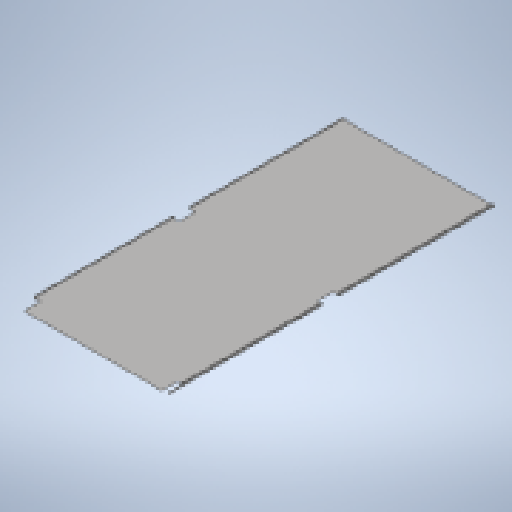
# Autodesk Inventor part: MSC 0101 sheet gills
Saved by Autodesk Inventor 2025 (Build 290162010, 162A)
## iProperties
Created: 2024-06-15
Part Number: MSC 0101 sheet gills
Material: Stainless Steel
Document SubType Name: Sheet Metal
Designer: pokla
Density: 8 g/cm^3
Sheet Metal Rule: Default_mm
Appearance: Default
Stock Number: МОО 0101 лист жабра
Mass: 7357.89 g
Surface Area: 36818.7 cm^2
Volume: 919.736 cm^3
Flat Pattern Width: 96.1524 cm
Flat Pattern Length: 200 cm
Flat Pattern Area: 19230.5 cm^2
Sheet Metal Width: 961,524 mm
Sheet Metal Length: 2000,000 mm
Sheet Metal Area: 1923047,787 mm^2
Author: pokla
Autodesk Inventor part; units mm, degrees
ref_plane "YZ Plane" through (0, 0, 0) normal (1, 0, 0) x (0, 1, 0)
ref_plane "XZ Plane" through (0, 0, 0) normal (0, 1, 0) x (-1, 0, 0)
ref_plane "XY Plane" through (0, 0, 0) normal (0, 0, 1) x (1, 0, 0)
sketch "Sketch6" plane through (0, 0, 0) normal (0, 1, 0) x (-1, 0, 0)
  line L0 (462.5, -1000) -> (-462.5, -1000)
  line L1 (-462.5, -1000) -> (-462.5, 1000)
  line L2 (-462.5, 1000) -> (462.5, 1000)
  line L3 (462.5, 1000) -> (462.5, -1000)
  line L4 (462.5, -1000) -> (-462.5, 1000) construction
  line L5 (-462.5, -1000) -> (462.5, 1000) construction
  point P0 (0, 0)
  dimension "d52" = 925
  dimension "d53" = 2000
  measures "d52" distance of L1.end L2.end
  measures "d53" distance of L0.end L1.end
extrude "Plate2" add sketch "Sketch6" along normal blind 0.5
sketch "Sketch10" plane through (-462, 0, 1000) normal (-1, 0, 0) x (0, -1, 0)
  line L0 (0, -2000) -> (0, 0)
  line L1 (0, 0) -> (-10, 0)
  line L2 (-10, 0) -> (-10, -2000)
  line L3 (-10, -2000) -> (0, -2000)
  constraints: 6 end point, 1 horizontal, 1 perpendicular, 1 vertical
edge flange "Flange1" height 10 angle 90 thickness 0.5 bend radius 0.5 thickness toward (-1, 0, 0) relief straight relief width 0.5 relief depth 0.25 corner gap 0.5 corner form 0 edges at (-462.5, 0.5, 0) (462.5, 0.5, 0) wall of the first edge with corners at (-462, 0, -1000) (-462, 0, 1000) (-462, 10, 1000) (-462, 10, -1000)
bend "Bend2"
corner "Corner2"
sketch "Sketch11" plane through (462.5, 9.5, -1000) normal (0, 1, 0) x (-1, 0, 0)
  line L0 (0, 2000) -> (0, 0)
  line L1 (0, 0) -> (10, 0)
  line L2 (10, 0) -> (10, 2000)
  line L3 (10, 2000) -> (0, 2000)
  constraints: 6 end point, 1 horizontal, 1 perpendicular, 1 vertical
edge flange "Flange2" height 10 angle 90 thickness 0.5 bend radius 0.5 thickness toward (0, 1, 0) relief straight relief width 0.5 relief depth 0.25 corner gap 0.5 corner form 0 edges at (462, 10, 0) (-462, 10, 0) wall of the first edge with corners at (462.5, 9.5, 1000) (462.5, 9.5, -1000) (452.5, 9.5, -1000) (452.5, 9.5, 1000)
bend "Bend3"
corner "Corner3"
sketch "Sketch12" plane through (0, 0, 0) normal (0, -1, 0) x (1, 0, 0)
  line L0 (462.5, -1000) -> (462.5, 1000) projected
  line L1 (462.5, 1000) -> (462.5, -1000) projected
  line L2 (-462.5, -1000) -> (-462.5, 1000) projected
  line L3 (-462.5, 1000) -> (-422.5, 1000)
  line L4 (-422.5, 1000) -> (-422.5, 900)
  line L5 (-422.5, 900) -> (-462.5, 900)
  line L6 (-462.5, 900) -> (-462.5, 1000)
  line L7 (-462.5, 15) -> (-422.5, 15)
  line L8 (-422.5, 15) -> (-422.5, -85)
  line L9 (-422.5, -85) -> (-462.5, -85)
  line L10 (-462.5, -85) -> (-462.5, 15)
  line L11 (462.5, 15) -> (422.5, 15)
  line L12 (422.5, 15) -> (422.5, -85)
  line L13 (422.5, -85) -> (462.5, -85)
  line L14 (462.5, -85) -> (462.5, 15)
  line L15 (461.5, -1000) -> (461.5, 1000) projected
  line L16 (462.5, 1000) -> (422.5, 1000)
  line L17 (422.5, 1000) -> (422.5, 900)
  line L18 (422.5, 900) -> (462.5, 900)
  line L19 (462.5, 900) -> (462.5, 1000)
  line L20 (-461.5, 1000) -> (461.5, 1000) projected
  point P0 (0, 0)
  point P1 (462.5, -85)
  point P2 (462.5, 15)
  point P3 (422.5, -35)
  point P4 (-422.5, -35)
  dimension "d96" = 100
  dimension "d97" = 40
  dimension "d100" = 100
  dimension "d101" = 40
  dimension "d102" = 100
  dimension "d103" = 40
  dimension "d105" = 1035
  dimension "d106" = 100
  dimension "d107" = 40
  dimension "d108" = 1035
  constraints: 32 end point, 8 parallel, 4 horizontal, 4 perpendicular, 2 midpoint, 2 point on line
  measures "d96" distance of L3.end L4.end
  measures "d97" distance of L2.end L3.end
  measures "d100" distance of L7.end L8.end
  measures "d101" distance of L7.start L7.end
  measures "d102" distance of L11.end L12.end
  measures "d103" distance of L11.start L11.end
  measures "d105" distance from line of L3 point (-422.5, -35)
  measures "d106" distance of L16.end L17.end
  measures "d107" distance of L1.start L16.end
  measures "d108" distance from line of L20 point (422.5, -35)
extrude "Extrusion3" cut sketch "Sketch12" against normal through all contours L13 L15 L11 L0 | L13 L12 L11 L15 | L18 L15 L16 L0 | L18 L17 L16 L15 | L2 L7 L8 L9 | L2 L3 L4 L5
equation "\"d105\" = d104"
equation "\"d52\" = ЖАБРЫ_базовая_ширина"
equation "\"d53\" = ЖАБРЫ_базовая_длина_дл_лист"
equation "\"d100\" = d96"
equation "\"d101\" = d97"
equation "\"d102\" = d98"
equation "\"d103\" = d97"
equation "\"d106\" = d96"
equation "\"d107\" = d97"
equation "\"d54\" = Thickness"
equation "\"d74\" = BendReliefWidth"
equation "\"d75\" = BendReliefDepth"
equation "\"d76\" = MinimumRemnant"
equation "\"d77\" = TransitionRadius"
equation "\"d80\" = BendRadius"
equation "\"d81\" = CornerReliefSize"
equation "\"d82\" = GapSize"
equation "\"d83\" = JacobiRadiusSize"
equation "\"d84\" = BendReliefWidth"
equation "\"d85\" = BendReliefDepth"
equation "\"d86\" = MinimumRemnant"
equation "\"d87\" = TransitionRadius"
equation "\"d90\" = BendRadius"
equation "\"d91\" = CornerReliefSize"
equation "\"d92\" = GapSize"
equation "\"d93\" = JacobiRadiusSize"
equation "\"BendRadius\" = Thickness"
equation "\"BendReliefWidth\" = Thickness"
equation "\"BendReliefDepth\" = 0.5 * Thickness"
equation "\"CornerReliefSize\" = 4 * Thickness"
equation "\"MinimumRemnant\" = 2 * Thickness"
equation "\"TransitionRadius\" = BendRadius"
equation "\"JacobiRadiusSize\" = BendRadius"
equation "\"GapSize\" = Thickness"
equation "\"d98\" = d96"
equation "\"ЖАБРЫ_базовая_ширина\" = 925"
equation "\"ЖАБРЫ_базовая_длина_дл_лист\" = 2000"
equation "\"Thickness\" = 0.5"
equation "\"d104\" = 1035"
body "Solid2"
